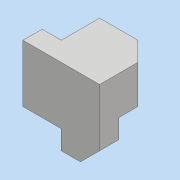
# Autodesk Inventor part: 10
Saved by Autodesk Inventor 2017 (Build 210142000, 142)
## iProperties
Part Number: 10
Material: 一般
Document SubType Name: Modeling
Designer: d8910
Density: 1 g/cm^3
Appearance: 預設
Author: d8910
Autodesk Inventor part; units mm, degrees
ref_plane "YZ Plane" through (0, 0, 0) normal (1, 0, 0) x (0, 1, 0)
ref_plane "XZ Plane" through (0, 0, 0) normal (0, 1, 0) x (-1, 0, 0)
ref_plane "XY Plane" through (0, 0, 0) normal (0, 0, 1) x (1, 0, 0)
sketch "草圖2" plane through (0, 0, 0) normal (0, 1, 0) x (-1, 0, 0)
  line L0 (10, 15) -> (-10, 15)
  line L1 (-10, 15) -> (-10, 0)
  line L2 (0, 0) -> (10, 0)
  line L3 (10, 0) -> (10, 15)
  line L4 (0, 0) -> (0, -5)
  line L5 (0, -5) -> (-5, -5)
  line L6 (-10, -5) -> (-10, -5) construction
  line L7 (-10, 0) -> (-5, -5)
  line L8 (-10, 0) -> (-10, -5) construction
  line L9 (-5, -5) -> (-10, -5) construction
  dimension "d6" = 5
  dimension "d7" = 15
  dimension "d8" = 20
  dimension "d9" = 10
  dimension "d10" = 20
  dimension "d11" = 5
  constraints: 20 end point, 4 parallel, 3 horizontal alignment, 2 perpendicular, 2 vertical alignment, 1 coincident, 1 horizontal
  measures "d6" distance of L2.start L4.end
  measures "d7" distance of L2.end L0.start
  measures "d8" distance of L0.start L0.end
  measures "d9" distance of L4.end L6.start
  measures "d10" distance of L0.end L6.end
  measures "d11" distance from line of L1 L5.end
extrude "擠出1" add sketch "草圖2" along normal blind 5
sketch "草圖3" plane through (-10, 0, 15) normal (0, 0, 1) x (1, 0, 0)
  line L0 (20, 0) -> (15, 0) construction
  line L1 (15, 0) -> (15, 5) construction
  line L2 (20, 5) -> (15, 5) construction
  line L3 (20, 0) -> (20, 5) construction
  line L4 (15, 0) -> (10, 0) construction
  line L5 (10, 0) -> (10, 5) construction
  line L6 (15, 5) -> (10, 5) construction
  line L7 (15, 0) -> (15, 5) construction
  line L8 (10, 0) -> (0, 0) construction
  line L9 (0, 0) -> (0, 5) construction
  line L10 (10, 5) -> (0, 5) construction
  line L11 (10, 0) -> (10, 5) construction
  line L12 (0, 5) -> (20, 5) projected
  line L13 (20, 5) -> (5, 5)
  line L14 (5, 5) -> (5, 15)
  line L15 (5, 15) -> (15, 15)
  line L16 (20, 10) -> (20, 5)
  line L17 (20, 10) -> (15, 15)
  dimension "d14" = 5
  dimension "d15" = 10
  dimension "d16" = 5
  dimension "d17" = 5
  constraints: 10 end point, 2 parallel, 1 horizontal, 1 perpendicular
  measures "d14" distance between parallel lines of L9 L14
  measures "d15" distance of L13.end L14.end
  measures "d16" distance from line of L16.start L15
  measures "d17" horizontal distance of L16.start L15.end
extrude "擠出2" add sketch "草圖3" against normal blind 10
